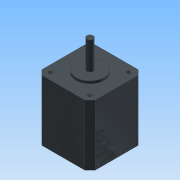
# Autodesk Inventor part: 42BYGHM809
Saved by Autodesk Inventor 2015 (Build 190159000, 159)
## iProperties
Created: 2013-12-24
Part Number: 42BYGHM809
Material: Iron, Cast
Document SubType Name: Modeling
Designer: aoki
Density: 1 g/cm^3
Appearance: Iron Gray
Author: aoki
Autodesk Inventor part; units mm, degrees
ref_plane "YZ Plane" through (0, 0, 0) normal (1, 0, 0) x (0, 1, 0)
ref_plane "XZ Plane" through (0, 0, 0) normal (0, 1, 0) x (-1, 0, 0)
ref_plane "XY Plane" through (0, 0, 0) normal (0, 0, 1) x (1, 0, 0)
sketch "Sketch1" plane through (0, 0, 0) normal (0, 0, 1) x (1, 0, 0)
  line L0 (21, 21) -> (-21, 21)
  line L1 (-21, 21) -> (-21, -21)
  line L2 (-21, -21) -> (21, -21)
  line L3 (21, -21) -> (21, 21)
  line L4 (21, 21) -> (-21, -21) construction
  line L5 (-21, 21) -> (21, -21) construction
  point P0 (0, 0)
  dimension "d0" = 42
  dimension "d1" = 42
  constraints: 12 end point, 2 midpoint, 2 parallel, 1 horizontal, 1 perpendicular
  measures "d0" distance of L2.end L1.end
  measures "d1" distance of L1.end L0.end
extrude "Extrusion1" add sketch "Sketch1" against normal blind 48
chamfer "Chamfer1" distance 4 angle 45 1 edges at (21, 21, -24)
chamfer "Chamfer2" distance 4 angle 45 2 edges at (21, -21, -24) (-21, 21, -24)
chamfer "Chamfer3" distance 4 angle 45 1 edges at (-21, -21, -24)
sketch "Sketch2" plane through (0, 0, 0) normal (0, 0, 1) x (1, 0, 0)
  circle A0 centre (0, 0) radius 11
  dimension "d13" = 22
  constraints: 1 centre point, 1 coincident
  measures "d13" diameter of A0
extrude "Extrusion2" add sketch "Sketch2" along normal blind 2
sketch "Sketch3" plane through (0, 0, 2) normal (0, 0, 1) x (1, 0, 0)
  circle A0 centre (0, 0) radius 11 projected
  circle A1 centre (0, 0) radius 2.5
  dimension "d16" = 5
  constraints: 1 centre point, 1 coincident
  measures "d16" diameter of A1
extrude "Extrusion3" add sketch "Sketch3" along normal blind 22 contours A1
sketch "Sketch4" plane through (0, 0, 0) normal (0, 0, 1) x (1, 0, 0)
  circle A0 centre (0, 0) radius 11 projected
  line L0 (-17, -21) -> (-21, -17) projected
  line L1 (-17, -21) -> (17, -21) projected
  line L2 (21, -17) -> (17, -21) projected
  line L3 (21, -17) -> (21, 17) projected
  line L4 (17, 21) -> (21, 17) projected
  line L5 (17, 21) -> (-17, 21) projected
  line L6 (-21, 17) -> (-17, 21) projected
  line L7 (-21, 17) -> (-21, -17) projected
  line L8 (0, -29.4) -> (0, 29.4) projected
  line L9 (-29.4, 0) -> (29.4, 0) projected
  point P0 (-15.5, 15.5)
  point P1 (15.5, 15.5)
  point P2 (-15.5, -15.5)
  point P3 (15.5, -15.5)
  dimension "d19" = 31
  dimension "d20" = 31
  constraints: 3 symmetric about line
  measures "d19" distance of point (15.5, 15.5) point (-15.5, 15.5)
  measures "d20" distance of point (-15.5, -15.5) point (-15.5, 15.5)
hole "Hole1" at (-15.5, 15.5, 0) at (15.5, 15.5, 0) at (-15.5, -15.5, 0) at (15.5, -15.5, 0) direction (0, 0, -1) diameter 3.242 depth 4 tip angle 118 thread size "M4x0.7" class "6H" standard "ANSI Metric M Profile"
body "Solid1"
